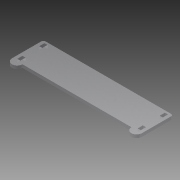
# Autodesk Inventor part: BackPanel
Saved by Autodesk Inventor 2015 SP1 (Build 190203100, 203)
## iProperties
Created: 2015-01-22
Part Number: BackPanel
Material: Acrylic, Clear
Document SubType Name: Modeling
Designer: Patrick
Density: 1.19 g/cm^3
Appearance: Transparent - Clear
Author: Patrick
Autodesk Inventor part; units mm, degrees
ref_plane "YZ Plane" through (0, 0, 0) normal (1, 0, 0) x (0, 1, 0)
ref_plane "XZ Plane" through (0, 0, 0) normal (0, 1, 0) x (-1, 0, 0)
ref_plane "XY Plane" through (0, 0, 0) normal (0, 0, 1) x (1, 0, 0)
sketch "Sketch1" plane through (0, 0, 0) normal (0, 0, 1) x (1, 0, 0)
  line L0 (-62, 15) -> (62, 15)
  line L1 (62, 15) -> (62, -15)
  line L2 (62, -15) -> (-62, -15)
  line L3 (-62, -15) -> (-62, 15)
  line L4 (-62, 15) -> (62, -15) construction
  line L5 (62, 15) -> (-62, -15) construction
  point P0 (0, 0)
  dimension "d0" = 124
  dimension "d1" = 30
  constraints: 12 end point, 2 midpoint, 2 parallel, 1 horizontal, 1 perpendicular
  measures "d0" distance of L1.end L2.end
  measures "d1" distance of L0.end L1.end
extrude "Extrusion1" add sketch "Sketch1" along normal blind 3
sketch "Sketch3" plane through (0, 0, 3) normal (0, 0, 1) x (1, 0, 0)
  line L0 (62, 15) -> (-62, 15) projected
  line L1 (-62, -15) -> (62, -15) projected
  arc A0 (-62, -15) -> (-52, -15) centre (-57, -15) ccw
  line L2 (-62, -15) -> (-52, -15)
  point P0 (0, 0)
  constraints: 2 end point, 2 point on circle, 1 centre point, 1 collinear, 1 point on line
extrude "Extrusion3" add sketch "Sketch3" against normal blind 3
mirror "Mirror2" about plane through (0, 0, 0) normal (1, 0, 0) of "Extrusion3"
fillet "Fillet1" radius 2 1 edges at (-62, 15, 1.5)
fillet "Fillet2" radius 2 1 edges at (62, 15, 1.5)
sketch "Sketch5" plane through (0, 0, 3) normal (0, 0, 1) x (1, 0, 0)
  line L0 (-58.96, 12.985) -> (-56.04, 12.985)
  line L1 (-56.04, 12.985) -> (-56.04, 8.015)
  line L2 (-56.04, 8.015) -> (-58.96, 8.015)
  line L3 (-58.96, 8.015) -> (-58.96, 12.985)
  line L4 (-58.96, 12.985) -> (-56.04, 8.015) construction
  line L5 (-56.04, 12.985) -> (-58.96, 8.015) construction
  line L6 (60, 15) -> (-60, 15) projected
  line L7 (-58.96, -8.015) -> (-56.04, -8.015)
  line L8 (-56.04, -8.015) -> (-56.04, -12.985)
  line L9 (-56.04, -12.985) -> (-58.96, -12.985)
  line L10 (-58.96, -12.985) -> (-58.96, -8.015)
  line L11 (-58.96, -8.015) -> (-56.04, -12.985) construction
  line L12 (-56.04, -8.015) -> (-58.96, -12.985) construction
  line L13 (-52, -15) -> (52, -15) projected
  point P0 (0, 0)
  point P1 (-57.5, 10.5)
  point P2 (-57.5, -10.5)
  point P3 (-57.5, -10.5)
  point P4 (-57.5, 10.5)
  dimension "d31" = 2.92
  dimension "d32" = 4.97
  dimension "d33" = 57.5
  dimension "d34" = 4.5
  dimension "d35" = 4.5
  dimension "d4" = 3
  dimension "d5" = 5
  dimension "d6" = 56
  dimension "d7" = 2
  dimension "d10" = 5
  dimension "d11" = 2
  constraints: 24 end point, 6 midpoint, 4 parallel, 2 equal length, 2 horizontal, 2 perpendicular, 1 vertical alignment
  measures "d31" distance of L1.end L2.end
  measures "d32" distance of L2.end L0.start
  measures "d33" horizontal distance of point (-57.5, 10.5) point (0, 0)
  measures "d34" distance from line of point (-57.5, 10.5) L6
  measures "d35" distance from line of point (-57.5, -10.5) L13
extrude "Extrusion5" cut sketch "Sketch5" against normal through all
mirror "Mirror3" about plane through (0, 0, 0) normal (1, 0, 0) of "Extrusion5"
equation "\"d35\" = d34"
equation "\"kerf\" = 0.13"
body "Solid1"
